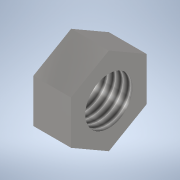
# Autodesk Inventor part: KOGANEI_unkown_35_M5Nut
Saved by Autodesk Inventor 2022.3 (Build 263350000, 350)
## iProperties
Created: 2022-04-18
Part Number: KOGANEI_unkown_35_M5Nut
Material: ステンレス鋼 440C
Document SubType Name: Modeling
Designer: YusukeKunita
Density: 7.75 g/cm^3
Appearance: 半つや出し
Author: YusukeKunita
Autodesk Inventor part; units mm, degrees
ref_plane "YZ Plane" through (0, 0, 0) normal (1, 0, 0) x (0, 1, 0)
ref_plane "XZ Plane" through (0, 0, 0) normal (0, 1, 0) x (-1, 0, 0)
ref_plane "XY Plane" through (0, 0, 0) normal (0, 0, 1) x (1, 0, 0)
sketch "スケッチ1" plane through (0, 0, 0) normal (0, 1, 0) x (-1, 0, 0)
  line L0 (0, 4.6188) -> (4, 2.3094)
  line L1 (-4, 2.3094) -> (0, 4.6188)
  line L2 (-4, -2.3094) -> (-4, 2.3094)
  line L3 (0, -4.6188) -> (-4, -2.3094)
  line L4 (4, -2.3094) -> (0, -4.6188)
  line L5 (4, 2.3094) -> (4, -2.3094)
  point P0 (0, 0)
  point P1 (0, 0)
  point P2 (0, 4.6188)
  point P3 (0, -4.6188)
  dimension "d2" = 360
  dimension "d4" = 8
  constraints: 12 end point, 2 coincident, 1 vertical alignment, 19 other
  measures "d4" distance between parallel lines of L5 L2
extrude "押し出し1" add sketch "スケッチ1" along normal blind 4
sketch "スケッチ2" plane through (0, 4, 0) normal (0, 1, 0) x (1, 0, 0)
  point P0 (0, 0)
  point P1 (0, 0)
  constraints: 1 coincident
hole "穴1" at (0, 4, 0) direction (0, -1, 0) diameter 5 end through all
thread "ねじ1" size "M5x0.8" class "6H" standard "ANSI Metric M Profile" full length
